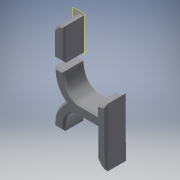
# Autodesk Inventor part: literak
Saved by Autodesk Inventor 2019 (Build 230136000, 136)
## iProperties
Created: 2020-10-14
Part Number: literak
Material: Ogólny
Document SubType Name: Modeling
Designer: Dawid
Density: 1 g/cm^3
Appearance: Domyślna
Author: Dawid
Autodesk Inventor part; units mm, degrees
ref_plane "YZ Plane" through (0, 0, 0) normal (1, 0, 0) x (0, 1, 0)
ref_plane "XZ Plane" through (0, 0, 0) normal (0, 1, 0) x (-1, 0, 0)
ref_plane "XY Plane" through (0, 0, 0) normal (0, 0, 1) x (1, 0, 0)
sketch "Szkic1" plane through (0, 0, 0) normal (0, 0, 1) x (1, 0, 0)
  line L0 (-1.7761, 3.0574) -> (3.9588, 3.0693)
  spline S0 degree 4 poles (-6.0129, 9.2984) (-6.0122, 8.8126) (-5.91, 7.8998) (-5.6765, 6.7488) (-5.0601, 5.4526) (-4.3689, 4.2263) (-3.1004, 3.6091) (-2.5574, 3.1452) (-1.7761, 3.0574) knots 0 0 0 0 0 0.302744 0.429487 0.556977 0.683363 1 1 1 1 1
  line L1 (-9.0161, 9.3008) -> (-6.0129, 9.2984)
  spline S1 degree 4 poles (-5.6394, 1.6539) (-6.2253, 2.0519) (-6.8441, 2.7086) (-7.5504, 3.6464) (-8.1909, 4.9461) (-8.6952, 6.3594) (-8.9286, 7.605) (-9.0078, 8.7103) (-9.0161, 9.3008) knots 0 0 0 0 0 0.30881 0.43146 0.555789 0.682893 1 1 1 1 1
  spline S2 degree 4 poles (-9.0159, -6.5073) (-8.9946, -5.9444) (-9.0506, -5.0193) (-8.8921, -3.8712) (-8.4467, -2.4724) (-7.779, -1.0175) (-6.9941, 0.1443) (-6.2441, 1.0282) (-5.6394, 1.6539) knots 0 0 0 0 0 0.292648 0.413818 0.537385 0.66449 1 1 1 1 1
  line L2 (-5.9717, -6.5073) -> (-9.0159, -6.5073)
  spline S3 degree 4 poles (-1.8711, -0.2267) (-2.4598, -0.2272) (-3.2295, -0.3454) (-4.0941, -0.7561) (-4.8987, -1.6476) (-5.5845, -2.8998) (-5.8796, -4.2669) (-5.9715, -5.5126) (-5.9717, -6.5073) knots 0 0 0 0 0 0.285173 0.397982 0.515184 0.640757 1 1 1 1 1
  line L3 (4.07, -0.2226) -> (-1.8711, -0.2267)
  line L4 (4.07, -8.0305) -> (4.07, -0.2226)
  spline S4 degree 4 poles (6.9436, -10.6857) (6.8295, -10.6721) (6.3962, -10.6081) (6.0064, -10.4424) (5.4067, -10.0768) (4.908, -9.5754) (4.4162, -8.9914) (4.0841, -8.4941) (4.07, -8.0305) knots 0 0 0 0 0 0.262174 0.383058 0.509233 0.642493 1 1 1 1 1
  line L5 (6.9176, 7.0884) -> (6.9436, -10.6857)
  spline S5 degree 4 poles (3.9588, 5.8479) (4.1949, 5.8112) (4.4622, 5.8281) (4.9879, 5.8903) (5.5271, 6.066) (6.0669, 6.3139) (6.4575, 6.6009) (6.7361, 6.8717) (6.9176, 7.0884) knots 0 0 0 0 0 0.298431 0.42419 0.551944 0.678948 1 1 1 1 1
  line L6 (3.9588, 3.0693) -> (3.9588, 5.8479)
  point P0 (-6.4798, 2.3682)
  point P1 (-7.1378, 3.1511)
  point P2 (-7.6971, 4.0062)
  point P3 (-8.1599, 4.9385)
  point P4 (-8.5262, 5.9545)
  point P5 (-8.7941, 7.0615)
  point P6 (-8.9593, 8.2671)
  point P7 (-5.9587, 8.4814)
  point P8 (-5.7853, 7.452)
  point P9 (-5.4824, 6.4248)
  point P10 (-5.0467, 5.4625)
  point P11 (-4.4781, 4.6134)
  point P12 (-3.6388, 3.9119)
  point P13 (-2.7914, 3.3839)
  point P14 (4.2948, 5.8276)
  point P15 (4.6657, 5.8611)
  point P16 (5.1126, 5.9452)
  point P17 (5.5268, 6.077)
  point P18 (5.9119, 6.2558)
  point P19 (6.2707, 6.4824)
  point P20 (6.6055, 6.7588)
  point P21 (-9.0067, -5.5778)
  point P22 (-8.9463, -4.5502)
  point P23 (-8.7553, -3.5291)
  point P24 (-8.4306, -2.5086)
  point P25 (-7.966, -1.4836)
  point P26 (-7.3529, -0.45)
  point P27 (-6.5812, 0.5953)
  point P28 (-2.8094, -0.3198)
  point P29 (-3.5995, -0.5864)
  point P30 (-4.2679, -1.0198)
  point P31 (-4.8324, -1.6312)
  point P32 (-5.2978, -2.4473)
  point P33 (-5.6559, -3.505)
  point P34 (-5.8884, -4.8449)
  point P35 (6.7095, -10.6489)
  point P36 (6.2916, -10.5393)
  point P37 (5.8825, -10.3549)
  point P38 (5.4493, -10.0776)
  point P39 (5.0766, -9.7357)
  point P40 (4.6764, -9.2819)
  point P41 (4.2779, -8.7172)
  constraints: 14 end point, 54 other
extrude "Wyciągnięcie proste1" add sketch "Szkic1" along normal blind 6
chamfer "Faza1" distance 0.5 angle 45 13 edges at (-5.0229, 5.4178, 6) (1.0913, 3.0634, 6) (5.5606, 6.0904, 6) (3.9588, 4.4586, 6) (6.9306, -1.7986, 6) (4.07, -4.1266, 6) (5.2764, -9.9329, 6) (1.0994, -0.2247, 6) (-5.0394, -1.9458, 6) (-7.4938, -6.5073, 6) (-8.3422, -2.287, 6) (-8.1867, 5.0024, 6) (-7.5145, 9.2996, 6)
ref_plane "Płaszczyzna konstrukcyjna1" through (-7.2971, 15.9284, 0) normal (0, 0, 1) x (1, 0, 0)
sketch "Szkic2" plane through (-7.2971, 15.9284, 0) normal (0, 0, 1) x (1, 0, 0)
  line L0 (1.302, -4.1378) -> (-1.5549, -4.1378)
  line L1 (1.302, 4.932) -> (1.302, -4.1378)
  spline S0 degree 4 poles (-1.5549, 2.5751) (-1.4537, 2.9011) (-1.2779, 3.3198) (-0.9845, 3.7877) (-0.5206, 4.2386) (0.0094, 4.6073) (0.5227, 4.8048) (0.9648, 4.8961) (1.302, 4.932) knots 0 0 0 0 0 0.318087 0.440079 0.560951 0.682796 1 1 1 1 1
  line L2 (-1.5549, -4.1378) -> (-1.5549, 2.5751)
  point P0 (7.2971, -15.9284)
  point P1 (-1.359, 3.0924)
  point P2 (-1.1188, 3.5353)
  point P3 (-0.8361, 3.9113)
  point P4 (-0.5104, 4.2267)
  point P5 (-0.1391, 4.4859)
  point P6 (0.2825, 4.6906)
  point P7 (0.7605, 4.8403)
  constraints: 6 end point, 9 other
extrude "Wyciągnięcie proste2" add sketch "Szkic2" along normal blind 6
chamfer "Faza2" distance 0.5 angle 45 4 edges at (-8.8521, 15.1471, 6) (-5.9952, 16.3255, 6) (-7.4236, 11.7906, 6) (-7.8092, 20.1537, 6)
